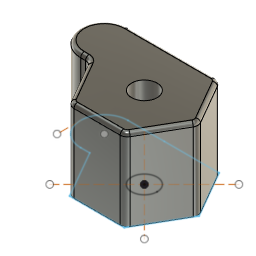
Adjustable_Bowden_Endstop (Autodesk Fusion 360 design; units mm, degrees)
Autodesk Fusion 360 part; units mm, degrees
sketch "Sketch1" plane through (0, 0, 0) normal (0, 0, 1) x (1, 0, 0)
  line L0 (6.5, 6.5) -> (-6.5, -6.5) construction
  line L1 (-6.5, 6.5) -> (6.5, -6.5) construction
  circle A0 centre (0, 0) radius 1.75
  line L2 (-6.5, 6.5) -> (-8.75, 6.5)
  arc A1 (-8.75, 6.5) -> (-8.75, 0) centre (-8.75, 3.25) ccw
  line L3 (-12, 3.25) -> (-12, 0) construction
  line L4 (7.5056, 0) -> (3.7528, 6.5)
  line L5 (3.7528, 6.5) -> (-3.7528, 6.5)
  line L6 (-7.5056, 0) -> (-3.7528, -6.5)
  line L7 (-3.7528, -6.5) -> (3.7528, -6.5)
  line L8 (3.7528, -6.5) -> (7.5056, 0)
  line L9 (-6.5, 6.5) -> (-3.7528, 6.5)
  line L10 (-8.75, 0) -> (-7.5056, 0)
  dimension "d1" = 13
  dimension "d2" = 13
  dimension "d3" = 3.5
  dimension "d8" = 12
  constraint coincident L0 A0.centre
  constraint coincident L1 A0.centre
  constraint coincident A0.centre origin
  constraint tangent L2 A1
  constraint midpoint A1 L3.start
  constraint tangent A1 L3
  constraint horizontal L7
  constraint parallel L5 L9
  constraint tangent A1 L10
  measures "d1" distance of L0.start L1.end
  measures "d2" distance of L0.start L1.start
  measures "d3" diameter of A0
  measures "d8" distance of A0.centre L3
extrude "Extrude3" add sketch "Sketch1" along normal blind 11.2
fillet "Fillet1" radius 1 5 edges at (-3.7528, -6.5, 5.6) (-7.5056, 0, 5.6) (3.7528, -6.5, 5.6) (7.5056, 0, 5.6) (3.7528, 6.5, 5.6)
fillet "Fillet2" radius 0.5 12 edges at (7.3509, 0, 11.2) (5.6292, 3.25, 11.2) (3.6754, 6.366, 11.2) (-2.7873, 6.5, 11.2) (-12, 3.25, 11.2) (-8.4165, 0, 11.2) (-7.5829, -0.134, 11.2) (-5.6292, -3.25, 11.2) (-3.6754, -6.366, 11.2) (0, -6.5, 11.2) (3.6754, -6.366, 11.2) (5.6292, -3.25, 11.2)
